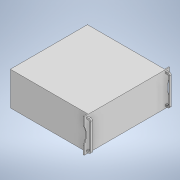
# Autodesk Inventor part: PC
Saved by Autodesk Inventor 2022 (Build 260153000, 153)
## iProperties
Created: 2022-08-18
Part Number: PC
Material: Generic
Document SubType Name: Modeling
Designer: Alok
Density: 1 g/cm^3
Appearance: Default
Author: Alok
Autodesk Inventor part; units mm, degrees
ref_plane "YZ Plane" through (0, 0, 0) normal (1, 0, 0) x (0, 1, 0)
ref_plane "XZ Plane" through (0, 0, 0) normal (0, 1, 0) x (-1, 0, 0)
ref_plane "XY Plane" through (0, 0, 0) normal (0, 0, 1) x (1, 0, 0)
sketch "Sketch1" plane through (0, 0, 0) normal (0, 1, 0) x (-1, 0, 0)
  line L0 (232.5, 230) -> (-232.5, 230)
  line L1 (-232.5, 230) -> (-232.5, -230)
  line L2 (-232.5, -230) -> (232.5, -230)
  line L3 (232.5, -230) -> (232.5, 230)
  line L4 (232.5, 230) -> (-232.5, -230) construction
  line L5 (-232.5, 230) -> (232.5, -230) construction
  point P0 (0, 0)
  dimension "d0" = 465
  dimension "d1" = 460
  constraints: 12 end point, 2 midpoint, 2 parallel, 1 horizontal, 1 perpendicular
  measures "d0" distance of L2.end L1.end
  measures "d1" distance of L1.end L0.end
extrude "Extrusion1" add sketch "Sketch1" along normal blind 200
sketch "Sketch3" plane through (232.5, 0, -230) normal (0, 0, -1) x (-1, 0, 0)
  line L0 (0, 0) -> (0, 200) projected
  line L1 (0, 200) -> (5, 200)
  line L2 (0, 200) -> (465, 200) projected
  line L3 (5, 200) -> (5, 0)
  line L4 (5, 0) -> (0, 0)
  line L5 (0, 0) -> (0, 200)
  point P0 (232.5, 0)
  dimension "d6" = 5
  constraints: 8 end point, 2 perpendicular, 1 parallel, 1 point on line
  measures "d6" distance of L0.end L1.end
extrude "Extrusion3" add sketch "Sketch3" along normal blind 25
sketch "Sketch4" plane through (-232.5, 0, 230) normal (0, 0, 1) x (1, 0, 0)
  line L0 (465, 0) -> (465, 200) projected
  line L1 (465, 200) -> (465, 0)
  line L2 (465, 0) -> (460, 0)
  line L3 (0, 0) -> (465, 0) projected
  line L4 (460, 0) -> (460, 200)
  line L5 (0, 200) -> (465, 200) projected
  point P0 (232.5, 0)
  dimension "d10" = 5
  constraints: 6 end point, 2 point on line, 1 collinear, 1 perpendicular
  measures "d10" distance of L0.start L2.end
extrude "Extrusion4" add sketch "Sketch4" along normal blind 25
sketch "Sketch5" plane through (232.5, 0, -255) normal (1, 0, 0) x (0, 0, -1)
  line L0 (-510, 100) -> (0, 100)
  line L1 (0, 200) -> (0, 0) projected
  line L2 (-510, 100) -> (-510, 150)
  line L3 (-510, 0) -> (-510, 200) projected
  line L4 (-510, 100) -> (-510, 50)
  line L5 (-510, 100) -> (-460, 100) construction
  arc A0 (-510, 50) -> (-510, 150) centre (-596.6025, 100) ccw
  line L6 (0, 100) -> (0, 150)
  line L7 (0, 100) -> (0, 50)
  arc A1 (0, 150) -> (0, 50) centre (86.6025, 100) ccw
  point P0 (-255, 0)
  point P1 (-510, 50)
  dimension "d13" = 50
  dimension "d14" = 50
  dimension "d15" = 90
  dimension "d16" = 100
  dimension "d17" = 50
  dimension "d18" = 100
  constraints: 12 end point, 4 point on circle, 3 point on line, 2 centre point, 1 collinear, 1 horizontal, 1 midpoint, 1 perpendicular
  measures "d13" distance of L0.start L2.end
  measures "d14" distance of L0.start L4.end
  measures "d15" angle of L4 L5
  measures "d16" radius of A0
  measures "d17" distance of L0.end L6.end
  measures "d18" radius of A1
extrude "Extrusion5" cut sketch "Sketch5" against normal blind 25
sketch "Sketch6" plane through (232.5, 0, 255) normal (1, 0, 0) x (0, 0, -1)
  line L0 (25, 0) -> (25, 200) projected
  line L1 (25, 190) -> (25, 180)
  line L2 (25, 180) -> (15, 180)
  line L3 (15, 180) -> (15, 190)
  line L4 (15, 190) -> (25, 190)
  point P0 (255, 0)
  point P1 (0, 200)
  dimension "d22" = 10
  dimension "d23" = 10
  constraints: 8 end point, 2 horizontal, 2 point on line
  measures "d22" distance of L1.start L1.end
  measures "d23" distance of L1.end L2.end
extrude "Extrusion6" add sketch "Sketch6" along normal blind 25
mirror "Mirror1" about plane through (0, 0, 0) normal (0, 0, 1) of "Extrusion6"
sketch "Sketch7" plane through (232.5, 0, 255) normal (1, 0, 0) x (0, 0, -1)
  line L0 (0, 0) -> (510, 0) projected
  line L1 (0, 50) -> (0, 0) projected
  line L2 (25, 0) -> (25, 200) projected
  line L3 (25, 10) -> (25, 20)
  line L4 (25, 20) -> (15, 20)
  line L5 (15, 20) -> (15, 10)
  line L6 (15, 10) -> (25, 10)
  point P0 (255, 0)
  dimension "d27" = 10
  dimension "d28" = 10
  constraints: 8 end point, 2 point on line, 1 horizontal, 1 perpendicular
  measures "d27" distance of L3.start L3.end
  measures "d28" distance of L3.end L4.end
extrude "Extrusion7" add sketch "Sketch7" along normal blind 25
mirror "Mirror2" about plane through (0, 0, 0) normal (0, 0, 1) of "Extrusion7"
sketch "Sketch8" plane through (232.5, 20, 240) normal (0, 1, 0) x (1, 0, 0)
  line L0 (25, 10) -> (25, 0) projected
  line L1 (25, 0) -> (25, 10)
  line L2 (25, 10) -> (20, 10)
  line L3 (0, 10) -> (25, 10) projected
  line L4 (20, 10) -> (20, 0)
  line L5 (0, 0) -> (25, 0) projected
  line L6 (25, 0) -> (20, 0)
  point P0 (-232.5, 240)
  dimension "d31" = 5
  dimension "d32" = 90
  constraints: 8 end point, 2 collinear, 1 perpendicular, 1 point on line, 1 vertical
  measures "d31" distance of L0.start L2.end
  measures "d32" angle of L2 L1
extrude "Extrusion8" add sketch "Sketch8" along normal blind 160
mirror "Mirror3" about plane through (0, 0, 0) normal (0, 0, 1) of "Extrusion8"
fillet "Face Fillet1" radius 10 1 edges at (252.5, 20, 235)
fillet "Face Fillet2" radius 10 1 edges at (257.5, 10, 235)
fillet "Face Fillet3" radius 10 1 edges at (257.5, 10, -235)
fillet "Face Fillet4" radius 10 1 edges at (257.5, 190, -235)
fillet "Face Fillet5" radius 10 1 edges at (257.5, 190, 235)
fillet "Face Fillet6" radius 10 1 edges at (252.5, 20, -235)
fillet "Face Fillet7" radius 10 1 edges at (252.5, 180, -235)
fillet "Face Fillet8" radius 10 1 edges at (252.5, 180, 235)
body "Solid1"
